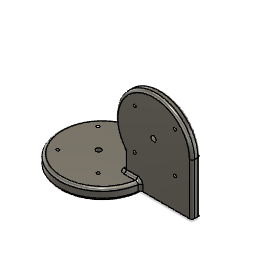
Cintura (Autodesk Fusion 360 design; units mm, degrees)
Autodesk Fusion 360 part; units mm, degrees
sketch "Sketch1" plane through (0, 0, 0) normal (0, 1, 0) x (1, 0, 0)
  circle A0 centre (0, 0) radius 50
  dimension "d1" = 100
  constraint coincident A0.centre origin
  measures "d1" diameter of A0
extrude "Extrude1" add sketch "Sketch1" along normal blind 10
sketch "Sketch2" plane through (0, 0, 0) normal (0, 1, 0) x (1, 0, 0)
  circle A0 centre (0, 0) radius 47.5
  dimension "d4" = 95
  constraint coincident A0.centre origin
  measures "d4" diameter of A0
extrude "Extrude2" add sketch "Sketch2" against normal blind 3
sketch "Sketch3" plane through (0, 0, 0) normal (0, 0, 1) x (1, 0, 0)
  line L0 (30, 0) -> (110, 0)
  line L1 (110, 0) -> (110, 50)
  line L2 (110, 50) -> (110, 60)
  arc A0 (110, 60) -> (30, 31.7157) centre (65, 60) ccw
  line L3 (30, 31.7157) -> (30, 0)
  dimension "d7" = 80
  dimension "d8" = 50
  dimension "d9" = 45
  dimension "d10" = 30
  dimension "d11" = 60
  constraint horizontal L0
  constraint perpendicular L0 L1
  constraint parallel L1 L2
  constraint tangent L2 A0
  constraint perpendicular L0 L3
  measures "d7" distance of L0.start L0.end
  measures "d8" distance of L0.end L1.end
  measures "d9" radius of A0
  measures "d10" distance of origin L0.start
  measures "d11" vertical distance of origin A0.centre
extrude "Extrude3" add sketch "Sketch3" along normal mid plane 10
sketch "Sketch4" plane through (0, 0, -5) normal (0, 0, -1) x (-1, 0, 0)
  line L0 (-49.7494, 10) -> (-30, 10)
  line L1 (-30, 10) -> (-30, 31.7157)
  arc A0 (-30, 31.7157) -> (-110, 60) centre (-65, 60) ccw
  line L2 (-110, 60) -> (-110, 0)
  line L3 (-110, 0) -> (-49.7494, 0)
  line L4 (-49.7494, 0) -> (-49.7494, 10)
  line L5 (-90, 82.244) -> (-42.756, 82.244)
  line L6 (-42.756, 82.244) -> (-42.756, 35)
  line L7 (-42.756, 35) -> (-90, 35)
  line L8 (-90, 35) -> (-90, 82.244)
  dimension "d14" = 47.244
  dimension "d15" = 47.244
  dimension "d16" = 25
  dimension "d17" = 25
  constraint horizontal L5
  constraint vertical L6
  constraint horizontal L7
  constraint vertical L8
  measures "d14" distance of L5.start L5.end
  measures "d15" distance of L5.start L7.end
  measures "d16" horizontal distance of A0.centre L7.end
  measures "d17" vertical distance of A0.centre L7.end
hole "Hole1" at (90, 82.244, -5) at (42.756, 82.244, -5) at (42.756, 35, -5) at (90, 35, -5) direction (0, 0, 1) diameter 3.332 end through all
hole "Hole2" at (65, 60, -5) direction (0, 0, 1) diameter 6 depth 10 tip angle 118
sketch "Sketch5" plane through (0, 10, 0) normal (0, 1, 0) x (-1, 0, 0)
  line L0 (-49.7494, 5) -> (-30, 5)
  line L1 (-30, 5) -> (-30, -5)
  line L2 (-30, -5) -> (-49.7494, -5)
  arc A0 (-49.7494, -5) -> (-49.7494, 5) centre (0, 0) ccw
  line L3 (30, -25) -> (-17.244, -25)
  line L4 (-17.244, -25) -> (-17.244, 22.244)
  line L5 (-17.244, 22.244) -> (30, 22.244)
  line L6 (30, 22.244) -> (30, -25)
  dimension "d24" = 47.244
  dimension "d25" = 47.244
  dimension "d26" = 30
  dimension "d27" = 25
  constraint horizontal L3
  constraint vertical L4
  constraint horizontal L5
  constraint vertical L6
  measures "d24" distance of L3.start L3.end
  measures "d25" distance of L3.start L5.end
  measures "d26" horizontal distance of A0.centre L3.start
  measures "d27" vertical distance of A0.centre L3.end
hole "Hole3" at (-30, 10, -25) at (17.244, 10, -25) at (17.244, 10, 22.244) at (-30, 10, 22.244) direction (0, -1, 0) diameter 3.332 depth 8 tip angle 118
thread "Thread1" "ISO Metric profile 4.0 M4x0.7 6H" major diameter 4.1095 minor diameter 3.332 pitch 0.7 angle 60 resizes the face on face at (16.1731, 7.3333, -26.2762) on face at (-31.0709, 7.3333, 20.9678) on face at (16.1731, 7.3333, 20.9678) on face at (-31.0709, 7.3333, -26.2762)
hole "Hole4" at (-5.9773, 10, -1.5751) direction (0, -1, 0) diameter 6 end through all
fillet "Fillet1" radius 3 1 edges at (-50, 10, 0)
fillet "Fillet2" radius 3 4 edges at (50, 102.4264, -5) (110, 30, -5) (110, 30, 5) (50, 102.4264, 5)
fillet "Fillet3" radius 3 2 edges at (30, 23.3918, -5) (30, 23.3918, 5)
fillet "Fillet4" radius 3 9 edges at (49.7494, 3.5, 5) (48.8635, 9.124, 5) (39.8666, 10, 5) (30.8787, 10, 4.1213) (30, 10, 0) (30.8787, 10, -4.1213) (39.8666, 10, -5) (48.8635, 9.124, -5) (49.7494, 3.5, -5)
